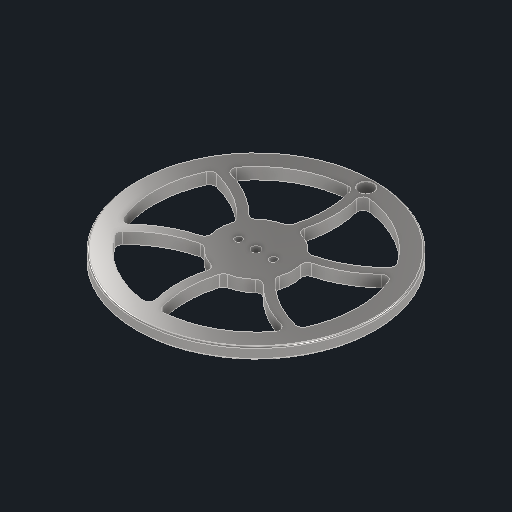
# Autodesk Inventor part: Wheel
Saved by Autodesk Inventor 2027.1 (Build 311270010, 270A)
## iProperties
Created: 2025-09-16
Material: Mild Steel S355 J2
Document SubType Name: Modeling
Designer: SD
Density: 7.85 g/cm^3
Appearance: Semi-Polished
Mass: 74.8165 g
Surface Area: 79.2261 cm^2
Volume: 9.53076 cm^3
Project: Automatic Tea Steeping mechanism
Part Number: Wheel
BOM-Mass: 0.07482
BOM-Area: 0.008
Thickness: 4.000 mm
Diameter: 82.500 mm
Procurement: Fabricate - 1st round
Build Stage: 2
Preferred Material: TBD
Author: SD
Title: Wheel
Autodesk Inventor part; units mm, degrees
ref_plane "YZ Plane" through (0, 0, 0) normal (1, 0, 0) x (0, 1, 0)
ref_plane "XZ Plane" through (0, 0, 0) normal (0, 1, 0) x (-1, 0, 0)
ref_plane "XY Plane" through (0, 0, 0) normal (0, 0, 1) x (1, 0, 0)
sketch "Sketch4" plane through (0, 0, 0) normal (0, 1, 0) x (-1, 0, 0)
  circle A0 centre (0, 0) radius 41.25
  constraints: 1 centre point, 1 coincident, 1 other
extrude "Extrusion2" add sketch "Sketch4" along normal mid plane 4
sketch "Sketch5" plane through (0, 2, 0) normal (0, 1, 0) x (1, 0, 0)
  circle A0 centre (0, 0) radius 35
  circle A1 centre (0, 0) radius 12.67
  dimension "d31" = 70
  dimension "d32" = 25.34
  constraints: 2 centre point, 2 coincident
  measures "d31" diameter of A0
  measures "d32" diameter of A1
extrude "Extrusion3" cut sketch "Sketch5" against normal through all
sketch "Sketch6" plane through (0, 2, 0) normal (0, 1, 0) x (1, 0, 0)
  circle A0 centre (0, 0) radius 12.67 projected
  arc A1 (-1.5, 12.5809) -> (-1.5, 34.9678) centre (-34.6618, 23.7744) ccw
  circle A2 centre (0, 0) radius 35 projected
  arc A3 (1.5, 12.5809) -> (1.5, 34.9678) centre (-31.6618, 23.7744) ccw
  dimension "d35" = 35
  dimension "d36" = 35
  dimension "d37" = 3
  dimension "d38" = 3
  dimension "d39" = 1.5
  constraints: 8 point on circle, 2 centre point, 1 vertical alignment
  measures "d35" radius of A1
  measures "d36" radius of A3
  measures "d37" distance of A2.end A1.end
  measures "d38" distance of A0.end A0.start
  measures "d39" horizontal distance of A1.end point (0, 0)
extrude "Extrusion4" add sketch "Sketch6" against normal blind 4 contours A0 A1 A2 A3 picked at (1.1323, 25.0378)
fillet "Fillet2" radius 2 4 edges at (-1.5, 0, -34.9678) (1.5, 0, -34.9678) (-1.5, 0, -12.5809) (1.5, 0, -12.5809)
pattern_circular "Circular Pattern1" count 6 over 360 about axis through (0, 0, 0) along (0, 1, 0) of "Extrusion4", "Fillet2"
fillet "Fillet3" radius 0.5 2 edges at (41.25, 2, 0) (41.25, -2, 0)
sketch "Sketch7" plane through (0, 2, 0) normal (0, 1, 0) x (1, 0, 0)
  point P0 (0, 0)
  point P1 (0, 0)
  point P2 (-6, 0)
  point P3 (6, 0)
  dimension "d47" = 6
  dimension "d48" = 12
  constraints: 2 horizontal alignment, 1 coincident
  measures "d47" distance of point (0, 0) point (-6, 0)
  measures "d48" distance of point (6, 0) point (-6, 0)
hole "Hole3" at (-6, 2, 0) at (6, 2, 0) direction (0, -1, 0) diameter 2.459 depth 8.8 thread size "M3x0.5" class "6H" standard "ISO Metric profile"
hole "Hole4" at (0, 2, 0) direction (0, -1, 0) diameter 3 depth 8.8
sketch "Sketch8" plane through (0, 2, 0) normal (0, 1, 0) x (1, 0, 0)
  circle A0 centre (0.5, 37.5) radius 2.5
  point P0 (0, 0)
  dimension "d63" = 5
  dimension "d64" = 37.5
  dimension "d65" = 0.5
  constraints: 1 centre point
  measures "d63" diameter of A0
  measures "d64" vertical distance of A0.centre point (0, 0)
  measures "d65" horizontal distance of point (0, 0) A0.centre
extrude "Extrusion5" cut sketch "Sketch8" against normal blind 10
chamfer "Chamfer1" distance 0.1 angle 45 2 edges at (-2, 2, -37.5) (-2, -2, -37.5)
equation "\"d36\" = d35"
body "Solid2"
